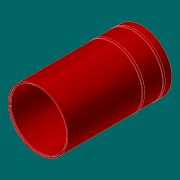
# Autodesk Inventor part: A1-19027-300-04 HCWI liner - nozzle
Saved by Autodesk Inventor 2017.3 (Build 213257000, 257)
## iProperties
Created: 2019-09-12
Part Number: A1-19027-300-04 HCWI liner - nozzle
Material: Iron, HCWI
Document SubType Name: Modeling
Designer: GVD
Density: 7.33517 g/cm^3
Appearance: Iron Gray(1)
Mass: 594290 g
Surface Area: 65077.3 cm^2
Volume: 81019.2 cm^3
Description: 28 1/2" ID x 1" WALL x 53 7/32" HCWI NOZZLE LINER, ASTM A532 CLASS III TYPE A, PF#(TBD)
Author: GVD
Autodesk Inventor part; units mm, degrees
ref_plane "YZ Plane" through (0, 0, 0) normal (1, 0, 0) x (0, 1, 0)
ref_plane "XZ Plane" through (0, 0, 0) normal (0, 1, 0) x (-1, 0, 0)
ref_plane "XY Plane" through (0, 0, 0) normal (0, 0, 1) x (1, 0, 0)
sketch "Sketch1" plane through (0, 0, 0) normal (0, 0, 1) x (1, 0, 0)
  circle A0 centre (0, 0) radius 361.95
  circle A1 centre (0, 0) radius 387.35
  dimension "d0" = 723.9
  dimension "d1" = 774.7
  constraints: 2 centre point, 2 coincident
  measures "d0" diameter of A0
  measures "d1" diameter of A1
extrude "Extrusion1" add sketch "Sketch1" along normal blind 1352
sketch "Sketch2" plane through (0, 0, 0) normal (0, 0, -1) x (-1, 0, 0)
  circle A0 centre (0, 0) radius 390.525
  circle A1 centre (0, 0) radius 387.35 projected
  dimension "d4" = 781.05
  constraints: 1 centre point, 1 coincident
  measures "d4" diameter of A0
extrude "Extrusion2" add sketch "Sketch2" against normal blind 114.3
fillet "Fillet1" radius 4.7625 1 edges at (-387.35, 0, 114.3)
ref_plane "Work Plane1" through (0, 0, 382) normal (0, 0, -1) x (-1, 0, 0)
sketch "Sketch3" plane through (0, 0, 382) normal (0, 0, -1) x (-1, 0, 0)
  circle A0 centre (0, 0) radius 391.8585
  circle A1 centre (0, 0) radius 387.35 projected
  dimension "d12" = 783.717
  constraints: 1 centre point, 1 coincident
  measures "d12" diameter of A0
extrude "Extrusion3" add sketch "Sketch3" along normal blind 25.4
sketch "Sketch4" plane through (0, 0, 0) normal (0, 0, -1) x (-1, 0, 0)
  circle A0 centre (0, 0) radius 390.525 projected
  circle A1 centre (0, 0) radius 387.5532
  dimension "d16" = 775.1064
  constraints: 1 centre point, 1 coincident
  measures "d16" diameter of A1
extrude "Extrusion4" cut sketch "Sketch4" against normal blind 88.9
sketch "Sketch5" plane through (0, 0, 1352) normal (0, 0, 1) x (1, 0, 0)
  circle A0 centre (0, 0) radius 374.65
  dimension "d20" = 749.3
  constraints: 1 centre point, 1 coincident
  measures "d20" diameter of A0
extrude "Extrusion5" cut sketch "Sketch5" against normal blind 12.7
fillet "Fillet2" radius 4.7625 2 edges at (-387.35, 0, 382) (-387.35, 0, 356.6)
fillet "Fillet3" radius 0.7937 2 edges at (387.5532, 0, 88.9) (-374.65, 0, 1339.3)
chamfer "Chamfer2" distance 0.7937 angle 45 1 edges at (-374.65, 0, 1352)
body "Solid1"
